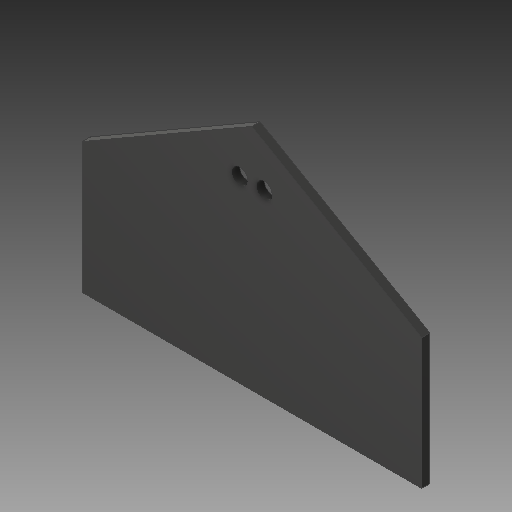
# Autodesk Inventor part: BA15
Saved by Autodesk Inventor 2017 (Build 210142000, 142)
## iProperties
Created: 2019-05-29
Part Number: BA15
Material: Wood (Cherry)
Document SubType Name: Modeling
Designer: Dell
Density: 0.63 g/cm^3
Appearance: Smooth - Black
Mass: 1160.74 g
Surface Area: 3116.93 cm^2
Volume: 1842.44 cm^3
Author: Dell
Autodesk Inventor part; units mm, degrees
ref_plane "YZ Plane" through (0, 0, 0) normal (1, 0, 0) x (0, 1, 0)
ref_plane "XZ Plane" through (0, 0, 0) normal (0, 1, 0) x (-1, 0, 0)
ref_plane "XY Plane" through (0, 0, 0) normal (0, 0, 1) x (1, 0, 0)
sketch "Sketch1" plane through (0, 0, 0) normal (0, 0, 1) x (1, 0, 0)
  line L0 (0, 0) -> (0, 201.9592)
  line L1 (0, 201.9592) -> (262.89, 353.7388)
  line L2 (262.89, 353.7388) -> (525.78, 201.9592)
  line L3 (525.78, 201.9592) -> (525.78, 0)
  line L4 (525.78, 0) -> (0, 0)
  point P0 (262.89, 0)
  dimension "d0" = 525.78
  dimension "d1" = 120
  dimension "d2" = 201.9592
  constraints: 10 end point, 1 horizontal alignment, 1 midpoint, 1 parallel, 1 perpendicular, 1 vertical, 1 vertical alignment
  measures "d0" distance of L3.end L0.start
  measures "d1" angle of L2 L1
  measures "d2" distance of L0.start L0.end
extrude "Extrusion1" add sketch "Sketch1" along normal blind 12.7
sketch "Sketch2" plane through (0, 0, 12.7) normal (0, 0, 1) x (1, 0, 0)
  circle A0 centre (243.84, 277.5388) radius 12.7
  circle A1 centre (281.94, 277.5388) radius 12.7
  line L0 (243.84, 277.5388) -> (281.94, 277.5388)
  point P0 (0, 0)
  point P1 (262.89, 277.5388)
  point P2 (262.89, 353.7388)
  dimension "d5" = 38.1
  dimension "d6" = 25.4
  dimension "d7" = 25.4
  dimension "d8" = 76.2
  constraints: 2 centre point, 2 end point, 1 horizontal, 1 midpoint, 1 vertical alignment
  measures "d5" distance of L0.start L0.end
  measures "d6" diameter of A1
  measures "d7" diameter of A0
  measures "d8" distance from line of point (262.89, 353.739) L0
extrude "Extrusion2" cut sketch "Sketch2" against normal through all
body "Solid1"
